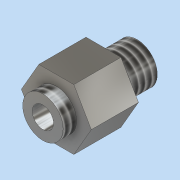
# Autodesk Inventor part: mainBody
Saved by Autodesk Inventor 2017 (Build 210142000, 142)
## iProperties
Created: 2016-10-25
Part Number: mainBody
Material: Nickel-Copper Alloy 400
Document SubType Name: Modeling
Designer: techn
Density: 8.83 g/cm^3
Appearance: Chrome - Polished
Author: techn
Autodesk Inventor part; units mm, degrees
ref_plane "YZ Plane" through (0, 0, 0) normal (1, 0, 0) x (0, 1, 0)
ref_plane "XZ Plane" through (0, 0, 0) normal (0, 1, 0) x (-1, 0, 0)
ref_plane "XY Plane" through (0, 0, 0) normal (0, 0, 1) x (1, 0, 0)
sketch "Sketch1" plane through (0, 0, 0) normal (0, 0, 1) x (1, 0, 0)
  line L0 (-5.1962, 0) -> (-2.5981, 4.5)
  line L1 (-2.5981, 4.5) -> (2.5981, 4.5)
  line L2 (2.5981, 4.5) -> (5.1962, 0)
  line L3 (5.1962, 0) -> (2.5981, -4.5)
  line L4 (2.5981, -4.5) -> (-2.5981, -4.5)
  line L5 (-2.5981, -4.5) -> (-5.1962, 0)
  point P0 (0, 0)
  point P1 (0, 0)
  dimension "d0" = 9
  constraints: 12 end point, 1 coincident, 13 other
  measures "d0" distance between parallel lines of L4 L1
extrude "Extrusion1" add sketch "Sketch1" along normal blind 7
sketch "Sketch2" plane through (0, 0, 7) normal (0, 0, 1) x (1, 0, 0)
  circle A0 centre (0, 0) radius 3
  dimension "d3" = 6
  constraints: 1 centre point, 1 coincident
  measures "d3" diameter of A0
extrude "Extrusion2" add sketch "Sketch2" along normal blind 2
sketch "Sketch3" plane through (0, 0, 0) normal (0, 0, -1) x (-1, 0, 0)
  circle A0 centre (0, 0) radius 3
  dimension "d6" = 6
  constraints: 1 centre point, 1 coincident
  measures "d6" diameter of A0
extrude "Extrusion3" add sketch "Sketch3" along normal blind 5
sketch "Sketch4" plane through (0, 0, 9) normal (0, 0, 1) x (1, 0, 0)
  circle A0 centre (0, 0) radius 1.585
  dimension "d9" = 3.17
  constraints: 1 centre point, 1 coincident
  measures "d9" diameter of A0
extrude "Extrusion4" cut sketch "Sketch4" against normal through all
thread "Thread1" size "M6x1" class "6g" standard "ANSI Metric M Profile" full length
thread "Thread2" size "M6x1" class "6g" standard "ANSI Metric M Profile" full length
body "Solid1"
